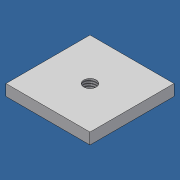
# Autodesk Inventor part: 093P45LN Back Plate
Saved by Autodesk Inventor 2012 (Build 160160000, 160)
## iProperties
Created: 2014-06-11
Part Number: 093P45LN Back Plate
Material: Aluminum-6061
Document SubType Name: Modeling
Designer: Mike Taylor
Mass: 32.3609 g
Surface Area: 51.8588 cm^2
Volume: 11.9413 cm^3
Density: 2.71 g/cm^3
Author: Mike Taylor
Autodesk Inventor part; units mm, degrees
ref_plane "YZ Plane" through (0, 0, 0) normal (1, 0, 0) x (0, 1, 0)
ref_plane "XZ Plane" through (0, 0, 0) normal (0, 1, 0) x (-1, 0, 0)
ref_plane "XY Plane" through (0, 0, 0) normal (0, 0, 1) x (1, 0, 0)
sketch "Sketch1" plane through (0, 0, 0) normal (0, 0, 1) x (1, 0, 0)
  line L0 (0, 0) -> (45, 0)
  line L1 (45, 0) -> (45, 6)
  line L2 (45, 6) -> (0, 6)
  line L3 (0, 6) -> (0, 0)
  dimension "d25" = 6
  dimension "d26" = 45
  constraints: 8 end point, 2 parallel, 1 horizontal, 1 perpendicular
  measures "d25" distance of L0.end L1.end
  measures "d26" distance of L1.end L2.end
extrude "Extrusion1" add sketch "Sketch1" along normal blind 45
sketch "Sketch5" plane through (0, 6, 0) normal (0, 1, 0) x (1, 0, 0)
  line L0 (45, 0) -> (45, -45) projected
  line L1 (45, 0) -> (0, 0) projected
  point P0 (22.5, -22.5)
  dimension "d27" = 22.5
  dimension "d28" = 22.5
  measures "d27" distance from line of point (22.5, -22.5) L0
  measures "d28" distance from line of L1 point (22.5, -22.5)
hole "Hole2" at (22.5, 6, 22.5) direction (0, -1, 0) diameter 6.6548 end through all
equation "\"d28\" = d27"
body "Solid1"
